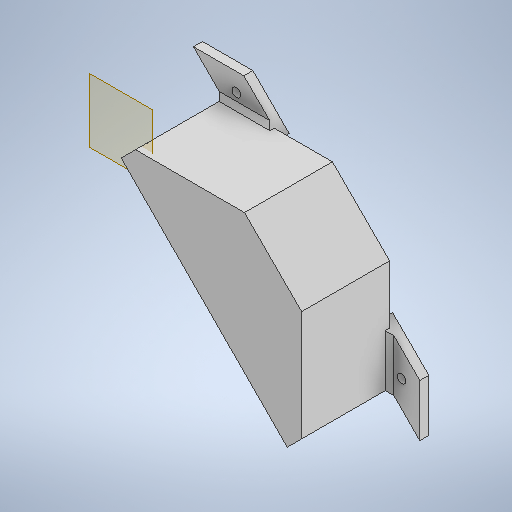
# Autodesk Inventor part: KimiRoofCover
Saved by Autodesk Inventor 2025.1 (Build 291241000, 241)
## iProperties
Created: 2026-05-07
Part Number: KimiRoofCover
Material: Generic
Document SubType Name: Modeling
Designer: User
Density: 1 g/cm^3
Appearance: Default
Author: User
## iProperties of the stored document KimiRoofCover_3DPrint.ipt
Created: 2026-05-07
Part Number: KimiRoofCover_3DPrint
Material: Generic
Document SubType Name: Modeling
Designer: User
Density: 1 g/cm^3
Appearance: Default
Author: User
Autodesk Inventor part; units mm, degrees
ref_plane "YZ Plane" through (0, 0, 0) normal (1, 0, 0) x (0, 1, 0)
sketch "Sketch1" plane through (0, 0, 0) normal (0, 0, 1) x (1, 0, 0)
  circle A0 centre (0, 12.272) radius 1.5 projected
  circle A1 centre (-56.8785, 69.1505) radius 1.5 projected
  line L0 (-54.2911, 75.397) -> (-41.7982, 62.9041) projected
  line L1 (-6.2464, 27.3523) -> (6.2464, 14.8594) projected
  line L2 (-54.2911, 75.397) -> (-96.5028, 75.397) projected
  line L3 (6.2464, -27.3523) -> (6.2464, 14.8594) projected
  line L4 (-69.4441, 75.397) -> (37.5985, 75.397) construction
  line L5 (-86.0099, 64.9041) -> (-40.9698, 64.9041) projected
  line L6 (-4.2464, 28.1807) -> (-4.2464, -16.8594) projected
  line L7 (-6.2464, 27.3523) -> (-6.2464, -14.8594)
  line L8 (-6.2464, 41.7773) -> (-6.2464, 27.3523)
  line L9 (-6.2464, 41.7773) -> (-6.2464, 27.3523)
  line L10 (-6.2464, 41.7773) -> (-27.3733, 62.9041)
  line L11 (-41.7982, 62.9041) -> (-27.3733, 62.9041)
  line L12 (-84.0099, 62.9041) -> (-41.7982, 62.9041)
  line L13 (-4.8322, 43.1915) -> (-26.5448, 64.9041)
  line L14 (-26.5448, 64.9041) -> (-41.7982, 64.9041)
  line L15 (-41.7982, 64.9041) -> (-84.0099, 64.9041)
  line L16 (-4.2464, 41.7773) -> (-4.2464, 27.3523)
  line L17 (-4.2464, 37.1495) -> (-4.2464, 42.6057)
  line L18 (-4.2464, 42.6057) -> (-4.8322, 43.1915)
  line L19 (-56.8785, 69.1505) -> (-61.125, 64.9041)
  line L20 (-56.8785, 69.1505) -> (-50.8731, 69.1505) construction
  line L21 (-71.6178, 75.397) -> (-59.2208, 62.9041)
  line L22 (-6.2464, 9.5204) -> (6.2464, -3.0691)
  dimension "d36" = 2
  dimension "d37" = 2
  dimension "d38" = 135
  constraints: 34 end point, 8 point on line, 4 horizontal, 3 vertical, 1 collinear, 1 equal length, 1 parallel, 9 other
  measures "d36" distance between parallel lines of L11 L14
  measures "d37" distance between parallel lines of L8 L16
  measures "d38" angle of L19 L20
ref_plane "Work Plane1" through (-54.2911, 14.8594, 3.1) normal (0, 0, 1) x (1, 0, 0)
extrude "Extrusion1" add sketch "Sketch1" along normal up to surface (3.1 mm away) contours L0 L5 L21 L2 | L0 L12 L21 L5 | L1 L6 L22 L7 | L1 L3 L22 L6
sketch "Sketch3" plane through (-6.3464, 41.7358, 0) normal (0.7071068, 0.7071068, 0) x (-0.7071068, 0.7071068, 0)
  line L0 (-0.0414, 3.1) -> (29.8364, 3.1) projected
  line L1 (-0.0414, 3.2) -> (29.8364, 3.2)
  line L2 (0, 0) -> (0, 3.1) projected
  line L3 (29.795, 0) -> (29.795, 3.1) projected
  line L4 (0, 3.2) -> (29.795, 3.2)
  line L5 (29.795, 3.2) -> (29.795, 5.2)
  line L6 (29.795, 5.2) -> (0, 5.2)
  line L7 (0, 5.2) -> (0, 3.2)
  point P0 (-33.9993, 0)
  point P1 (0, 8.1)
  point P2 (29.795, 8.1)
  point P3 (0, 5.2)
  point P4 (29.795, 3.2)
  point P5 (29.795, 3.2)
  dimension "d8" = 0.1
  dimension "d9" = 29.795
  dimension "d10" = 2
  constraints: 10 end point, 3 parallel, 3 point on line, 1 horizontal, 1 perpendicular
  measures "d8" distance between parallel lines of L0 L1
  measures "d9" distance of L6.end L5.end
  measures "d10" distance of L5.end L4.end
ref_plane "Work Plane2" through (-13.9814, 55.1691, -2.7) normal (0.7071068, 0.7071068, 0) x (-0.7071068, 0.7071068, 0)
extrude "Extrusion3" [suppressed]
ref_plane "Work Plane3" through (-68.3127, 66.8041, 31.3624) normal (0, 0, 1) x (1, 0, 0)
sketch "Sketch11" plane through (6.2464, -3.0691, 3.1) normal (0, 0, 1) x (1, 0, 0)
  line L0 (-12.4929, 44.8463) -> (-12.4929, 30.4214) projected
  line L1 (-12.4929, 30.4214) -> (0, 17.9285) projected
  line L2 (-10.4929, 31.2498) -> (-10.4929, 45.6748) projected
  line L3 (-10.3929, -12.2335) -> (-10.3929, 31.2912) projected
  line L4 (-10.3929, 45.4334) -> (-10.3929, 31.2912) projected
  line L5 (-10.3929, 45.4334) -> (-10.3929, 60.346) projected
  circle A0 centre (-2.9669, 29.4614) radius 1.5 projected
  circle A1 centre (-6.8189, 36.2632) radius 1.5 projected
  circle A2 centre (-42.2029, 71.6472) radius 1.5 projected
  circle A3 centre (-49.0047, 75.4992) radius 1.5 projected
  line L6 (2.7071, 35.3032) -> (-43.1629, 81.1732) projected
  line L7 (-43.1629, 81.1732) -> (-57.8305, 81.1732) projected
  line L8 (-57.8305, 81.1732) -> (-60.5376, 78.4661) projected
  line L9 (-60.5376, 78.4661) -> (-48.0447, 65.9732) projected
  line L10 (-48.0447, 65.9732) -> (-33.6197, 65.9732) projected
  line L11 (-12.4929, 44.8463) -> (-33.6197, 65.9732) projected
  line L12 (-12.4929, 44.8463) -> (-12.4929, 30.4214) projected
  line L13 (-12.4929, 30.4214) -> (0, 17.9285) projected
  line L14 (0, 17.9285) -> (2.7071, 20.6356) projected
  line L15 (2.7071, 20.6356) -> (2.7071, 35.3032) projected
  line L16 (-47.1748, 68.0732) -> (-33.0327, 68.0732) projected
  line L17 (-90.6995, 68.0732) -> (-47.1748, 68.0732) projected
  line L18 (-33.0327, 68.0732) -> (-18.0857, 68.0732) projected
  line L19 (-12.4929, 12.5894) -> (-12.4929, 30.4214) projected
  line L20 (0, 0) -> (-12.4929, 12.5894) projected
  line L21 (-48.0447, 65.9732) -> (-65.4672, 65.9732) projected
  line L22 (-65.4672, 65.9732) -> (-77.8643, 78.4661) projected
  point P0 (-6.2464, 3.0691)
  point P1 (-10.3929, 10.4732)
  point P2 (-10.3929, 48.4032)
  point P3 (-30.0629, 68.0732)
  point P4 (-67.5511, 68.0732)
extrude "Extrusion11" add sketch "Sketch11" along normal blind 10 contours L11 L10 L9 L17 L16 L18 L6 L5 L4 L3 L1 L0 | L1 L3 L20 L19 | L21 L22 L17 L9
sketch "Sketch12" plane through (6.2464, -3.0691, 13.1) normal (0, 0, 1) x (1, 0, 0)
  line L0 (-12.4929, 12.5894) -> (-10.3929, 10.4732) projected
  line L1 (-10.3929, 10.4732) -> (-10.3929, 48.4032) projected
  line L2 (-10.3929, 48.4032) -> (-30.0629, 68.0732) projected
  line L3 (-30.0629, 68.0732) -> (-67.5511, 68.0732) projected
  line L4 (-67.5511, 68.0732) -> (-65.4672, 65.9732) projected
  line L5 (-65.4672, 65.9732) -> (-33.6197, 65.9732) projected
  line L6 (-33.6197, 65.9732) -> (-12.4929, 44.8463) projected
  line L7 (-12.4929, 44.8463) -> (-12.4929, 12.5894) projected
  point P0 (-6.2464, 3.0691)
extrude "Extrusion12" add sketch "Sketch12" along normal up to surface (18.2624 mm away)
sketch "Sketch13" plane through (-61.3047, 65.0041, 31.3624) normal (0, 0, 1) x (1, 0, 0)
  line L0 (37.4882, 0) -> (57.1582, -19.67) projected
  line L1 (0, 0) -> (37.4882, 0) projected
  line L2 (57.1582, -19.67) -> (57.1582, -57.6) projected
  line L3 (0, 0) -> (-6.364, -6.364)
  line L4 (0, 0) -> (9, 0) construction
  line L5 (57.1582, -57.6) -> (50.7942, -63.9639)
  line L6 (57.1582, -57.6) -> (66.1582, -57.6) construction
  line L7 (50.7942, -63.9639) -> (-6.364, -6.364)
  point P0 (61.3047, -65.0041)
  dimension "d43" = 9
  dimension "d44" = 135
  dimension "d45" = 9
  dimension "d46" = 135
  constraints: 10 end point, 2 equal length, 2 horizontal
  measures "d43" distance of L1.start L3.end
  measures "d44" angle of L3 L4
  measures "d45" distance of L2.end L5.end
  measures "d46" angle of L5 L6
extrude "Extrusion13" add sketch "Sketch13" along normal blind 2
chamfer "Chamfer2" distance 2 angle 45 1 edges at (-39.0895, 29.8402, 33.3624)
chamfer "Chamfer3" distance 2 angle 45 2 edges at (-5.1964, 8.4623, 31.3624) (-60.2627, 63.9541, 31.3624)
chamfer "Chamfer4" distance 1.5 angle 45 2 edges at (-4.1464, 16.3282, 3.1) (-52.6015, 65.0041, 3.1)
body "Solid1"
